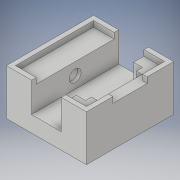
# Autodesk Inventor part: Enclosure_Bottom V1D6
Saved by Autodesk Inventor 2017 (Build 210142000, 142)
## iProperties
Created: 2018-02-12
Part Number: Enclosure_Bottom V1D6
Material: Generic
Document SubType Name: Modeling
Designer: Tripl_000
Density: 1 g/cm^3
Appearance: Default
Author: Tripl_000
Autodesk Inventor part; units mm, degrees
ref_plane "YZ Plane" through (0, 0, 0) normal (1, 0, 0) x (0, 1, 0)
ref_plane "XZ Plane" through (0, 0, 0) normal (0, 1, 0) x (-1, 0, 0)
ref_plane "XY Plane" through (0, 0, 0) normal (0, 0, 1) x (1, 0, 0)
sketch "Sketch1" plane through (0, 0, 0) normal (0, 1, 0) x (-1, 0, 0)
  line L0 (17.5, 19.05) -> (-17.5, 19.05)
  line L1 (-17.5, 19.05) -> (-17.5, -19.05)
  line L2 (-17.5, -19.05) -> (17.5, -19.05)
  line L3 (17.5, -19.05) -> (17.5, 19.05)
  line L4 (17.5, 19.05) -> (-17.5, -19.05) construction
  line L5 (-17.5, 19.05) -> (17.5, -19.05) construction
  point P0 (0, 0)
  dimension "d0" = 38.1
  dimension "d1" = 35
  constraints: 12 end point, 2 midpoint, 2 parallel, 1 horizontal, 1 perpendicular
  measures "d0" distance of L2.end L0.start
  measures "d1" distance between parallel lines of L1 L3
extrude "Extrusion1" add sketch "Sketch1" along normal blind 20
shell "Shell1" thickness 2 removed faces 1 at (5.8333, 20, -6.35)
sketch "Sketch2" plane through (-15.5, 2, 17.05) normal (0, 1, 0) x (1, 0, 0)
  line L0 (31, 34.1) -> (0, 34.1) projected
  line L1 (31, 0) -> (31, 34.1) projected
  line L2 (0, 34.1) -> (31, 34.1)
  line L3 (31, 34.1) -> (31, 0)
  line L4 (31, 0) -> (0, 0)
  line L5 (0, 0) -> (0, 34.1)
  point P0 (15.5, 17.05)
  constraints: 8 end point, 2 parallel, 1 horizontal, 1 perpendicular
extrude "Extrusion2" add sketch "Sketch2" along normal blind 15.5
sketch "Sketch3" plane through (0, 20, 0) normal (0, 1, 0) x (1, 0, 0)
  line L0 (17.5, 19.05) -> (-17.5, 19.05) projected
  line L1 (-17.5, -19.05) -> (17.5, -19.05) projected
  line L2 (0, 19.05) -> (-6.5, 19.05)
  line L3 (-6.5, 19.05) -> (-6.5, -19.05)
  line L4 (-6.5, -19.05) -> (0, -19.05)
  line L5 (0, -19.05) -> (0, 19.05)
  point P0 (0, 0)
  dimension "d7" = 6.5
  constraints: 8 end point, 2 parallel, 1 horizontal, 1 midpoint, 1 perpendicular, 1 point on line
  measures "d7" distance between parallel lines of L5 L3
extrude "Extrusion3" cut sketch "Sketch3" against normal blind 13
ref_plane "Work Plane1" through (0, 20, -19.05) normal (-1, 0, 0) x (0, 0, 1)
mirror "Mirror1" about plane through (0, 20, -19.05) normal (-1, 0, 0) of "Extrusion3"
sketch "Sketch4" plane through (-15.5, 17.5, 17.05) normal (0, 1, 0) x (1, 0, 0)
  line L0 (22, -2) -> (22, 36.1) projected
  line L1 (22, 17.05) -> (26, 17.05)
  line L2 (26, 17.05) -> (26, 29.55)
  line L3 (26, 29.55) -> (22, 29.55)
  line L4 (22, 29.55) -> (22, 17.05)
  point P0 (15.5, 17.05)
  dimension "d11" = 4
  dimension "d12" = 12.5
  constraints: 8 end point, 2 parallel, 1 horizontal, 1 midpoint, 1 perpendicular
  measures "d11" distance between parallel lines of L2 L0
  measures "d12" distance between parallel lines of L1 L3
extrude "Extrusion4" cut sketch "Sketch4" against normal up to surface (10.5 mm away)
sketch "Sketch5" plane through (-15.5, 17.5, 17.05) normal (0, 1, 0) x (1, 0, 0)
  line L0 (26, 17.05) -> (26, 29.55) projected
  line L1 (26, 17.05) -> (28.5, 17.05)
  line L2 (28.5, 17.05) -> (28.5, 26.85)
  line L3 (28.5, 26.85) -> (26, 26.85)
  line L4 (26, 26.85) -> (26, 17.05)
  point P0 (15.5, 17.05)
  dimension "d15" = 9.8
  dimension "d16" = 2.5
  constraints: 8 end point, 2 parallel, 1 horizontal, 1 perpendicular
  measures "d15" distance between parallel lines of L1 L3
  measures "d16" distance between parallel lines of L0 L2
extrude "Extrusion5" cut sketch "Sketch5" against normal blind 12.7
sketch "Sketch6" plane through (0, 20, 0) normal (0, 1, 0) x (1, 0, 0)
  line L0 (15.5, 17.05) -> (15.5, -17.05) projected
  line L1 (15.5, 0) -> (19.9746, 0)
  line L2 (19.9746, 0) -> (19.9746, 7.5)
  line L3 (19.9746, 7.5) -> (15.5, 7.5)
  line L4 (15.5, 7.5) -> (15.5, 0)
  point P0 (0, 0)
  dimension "d19" = 7.5
  constraints: 8 end point, 2 parallel, 1 horizontal, 1 midpoint, 1 perpendicular
  measures "d19" distance between parallel lines of L1 L3
extrude "Extrusion6" cut sketch "Sketch6" against normal up to surface (2.5 mm away)
ref_plane "Work Plane2" through (6.5, 7, 0) normal (0, 0, -1) x (-1, 0, 0)
mirror "Mirror2" about plane through (6.5, 7, 0) normal (0, 0, -1) of "Extrusion4", "Extrusion5", "Extrusion6"
sketch "Sketch7" plane through (-17.5, 0, -19.05) normal (-1, 0, 0) x (0, 0, 1)
  circle A0 centre (19.05, 12.14) radius 2.6
  line L0 (0, 20) -> (38.1, 20) projected
  point P0 (19.05, 0)
  dimension "d23" = 5.2
  dimension "d24" = 7.86
  constraints: 1 centre point
  measures "d23" diameter of A0
  measures "d24" distance from line of L0 A0.centre
extrude "Extrusion7" cut sketch "Sketch7" against normal up to surface (11 mm away)
sketch "Sketch8" plane through (-17.5, 0, -19.05) normal (-1, 0, 0) x (0, 0, 1)
  circle A0 centre (19.05, 12.14) radius 2.6 projected
  circle A1 centre (19.05, 12.14) radius 3.2
  point P0 (19.05, 0)
  dimension "d27" = 6.4
  constraints: 1 centre point, 1 coincident
  measures "d27" diameter of A1
extrude "Extrusion8" cut sketch "Sketch8" against normal blind 9.5
body "Solid1"
